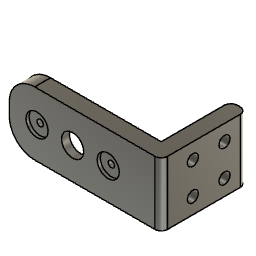
arm_1 v8 (Autodesk Fusion 360 design; units mm, degrees)
Autodesk Fusion 360 part; units mm, degrees
note: some values were not read from the file. Chosen so that the rebuilt part matches the saved one: which face or edge a step refers to.
sketch "스케치1" plane through (0, 0, 0) normal (0, 0, 1) x (1, 0, 0)
  line L0 (0, 0) -> (-45, 0)
  line L1 (-45, 0) -> (-45, 5)
  line L2 (-45, 5) -> (-5, 5)
  line L3 (0, 5) -> (0, 0)
  line L4 (0, 0) -> (-5, 0)
  line L5 (-5, 5) -> (-5, 30)
  line L6 (-5, 30) -> (0, 30)
  line L7 (0, 30) -> (0, 0)
  constraint horizontal L0
  constraint vertical L1
  constraint horizontal L2
  constraint vertical L3
  constraint coincident L0.start L3.end
  constraint horizontal L4
  constraint vertical L5
  constraint horizontal L6
  constraint vertical L7
extrude "돌출1" add sketch "스케치1" along normal blind 30
sketch "스케치2" plane through (0, 5, 0) normal (0, 1, 0) x (-1, 0, 0)
  circle A0 centre (25, 15) radius 7.5
  dimension "d3" = 15
  measures "d3" diameter of A0
extrude "돌출2" cut sketch "스케치2" against normal blind 2.5
sketch "스케치3" plane through (0, 5, 0) normal (0, 1, 0) x (-1, 0, 0)
  circle A0 centre (25, 15) radius 3.5
  dimension "d7" = 7
  measures "d7" diameter of A0
extrude "돌출3" cut sketch "스케치3" against normal blind 2.5 from surface at -2.5
sketch "스케치4" plane through (0, 5, 0) normal (0, 1, 0) x (-1, 0, 0)
sketch "스케치5" plane through (0, 0, 0) normal (0, -1, 0) x (1, 0, 0)
  circle A0 centre (-16.225, 15) radius 1
  dimension "d12" = 2
  measures "d12" diameter of A0
hole "구멍1" at (-16.225, 0, 15) direction (0, 1, 0) diameter 2 depth 7 tip angle 118
sketch "스케치6" plane through (0, 0, 0) normal (0, -1, 0) x (1, 0, 0)
hole "구멍2" at (-36.2538, 0, 15.3762) direction (0, 1, 0) diameter 2 depth 7 tip angle 118
delete_face "면 삭제1" 1 faces at (-16.1752, 1.6667, 14.0012)
sketch "스케치7" plane through (0, 0, 0) normal (0, -1, 0) x (1, 0, 0)
  circle A0 centre (-13.75, 15) radius 1
  dimension "d20" = 2
  measures "d20" diameter of A0
hole "구멍3" at (-13.75, 0, 15) direction (0, 1, 0) diameter 2 depth 7 tip angle 118
sketch "스케치8" plane through (0, 0, 0) normal (0, -1, 0) x (1, 0, 0)
delete_face "면 삭제2" 1 faces at (-35.9118, 1.6667, 16.3159)
delete_face "면 삭제3" 1 faces at (-13.7002, 1.6667, 14.0012)
sketch "스케치9" plane through (0, 0, 0) normal (0, -1, 0) x (1, 0, 0)
  circle A0 centre (-13.75, 15) radius 1
  dimension "d24" = 2
  measures "d24" diameter of A0
hole "구멍4" at (-13.75, 0, 15) direction (0, 1, 0) diameter 2 depth 7 tip angle 118
sketch "스케치10" plane through (0, 0, 0) normal (0, -1, 0) x (1, 0, 0)
  circle A0 centre (-36.25, 15) radius 1
  dimension "d28" = 2
  measures "d28" diameter of A0
hole "구멍5" at (-36.25, 0, 15) direction (0, 1, 0) diameter 2 depth 7 tip angle 118
sketch "스케치11" plane through (0, 0, 0) normal (0, -1, 0) x (1, 0, 0)
sketch "스케치12" plane through (0, 0, 0) normal (0, -1, 0) x (1, 0, 0)
sketch "스케치13" plane through (0, 0, 0) normal (0, -1, 0) x (1, 0, 0)
  circle A0 centre (-13.75, 15) radius 1
  circle A1 centre (-13.75, 15) radius 3.5
  dimension "d32" = 2
  dimension "d33" = 7
  constraint concentric A0 A1
  measures "d32" diameter of A0
  measures "d33" diameter of A1
extrude "돌출4" cut sketch "스케치13" against normal blind 1
sketch "스케치14" plane through (0, 0, 0) normal (0, -1, 0) x (1, 0, 0)
  circle A0 centre (-36.25, 15) radius 1
  circle A1 centre (-36.25, 15) radius 3.5
  dimension "d36" = 2
  dimension "d37" = 7
  constraint concentric A0 A1
  measures "d36" diameter of A0
  measures "d37" diameter of A1
extrude "돌출5" cut sketch "스케치14" against normal blind 1
sketch "스케치15" plane through (0, 0, 0) normal (1, 0, 0) x (0, 1, 0)
  circle A0 centre (20, 10) radius 1.75
  circle A1 centre (10, 10) radius 1.75
  circle A2 centre (20, 20) radius 1.75
  circle A3 centre (10, 20) radius 1.75
  dimension "d40" = 3.5
  dimension "d41" = 3.5
  dimension "d42" = 3.5
  dimension "d43" = 3.5
  measures "d40" diameter of A0
  measures "d41" diameter of A1
  measures "d42" diameter of A2
  measures "d43" diameter of A3
hole "구멍6" at (0, 20, 10) direction (-1, 0, 0) diameter 3.5 depth 7 tip angle 118
sketch "스케치16" plane through (0, 0, 0) normal (1, 0, 0) x (0, 1, 0)
  circle A0 centre (10, 10) radius 1.75
  dimension "d47" = 3.5
  measures "d47" diameter of A0
hole "구멍7" at (0, 10, 10) direction (-1, 0, 0) diameter 3.5 depth 7 tip angle 118
sketch "스케치17" plane through (0, 0, 0) normal (1, 0, 0) x (0, 1, 0)
  circle A0 centre (20, 20) radius 1.75
  dimension "d51" = 3.5
  measures "d51" diameter of A0
extrude "돌출6" cut sketch "스케치17" against normal blind 5
sketch "스케치18" plane through (0, 0, 0) normal (1, 0, 0) x (0, 1, 0)
  circle A0 centre (10, 20) radius 1.75
  dimension "d54" = 3.5
  measures "d54" diameter of A0
hole "구멍8" at (0, 10, 20) direction (-1, 0, 0) diameter 3.5 depth 7 tip angle 118
sketch "스케치19" plane through (0, 30, 0) normal (0, 1, 0) x (-1, 0, 0)
sketch "스케치20" plane through (0, 30, 0) normal (0, 1, 0) x (-1, 0, 0)
move_face "면 이동1" by (0, 0, 5) 1 faces at (-16.6667, 1.6667, 0)
move_face "면 이동2" by (0, 0, -5) 1 faces at (-16.6667, 1.6667, 30)
sketch "스케치24" plane through (0, 30, 0) normal (0, 1, 0) x (-1, 0, 0)
extrude "돌출7" cut 1 faces at (-3.3333, 30, 18.3333) along direction (0, -1, 0) blind 3
move_face "면 이동3" to x (1, 0, 0) y (0, 1, 0) z (0, 0, 1) at (-3, 0, 0) 3 faces at (-36.7283, 2.3333, 15.8782) (-33.5973, 1, 14.8012) (-32.7544, 0.6667, 14.8255)
move_face "면 이동4" to x (1, 0, 0) y (0, 1, 0) z (0, 0, 1) at (-3, 0, 0) 3 faces at (-28.4826, 0.8333, 14.6515) (-31.1257, 2.5, 14.4535) (-32.4907, 3.3333, 14.6262)
move_face "면 이동5" by (-3, 0, 0) 1 faces at (-45, 1.6667, 18.3333)
move_face "면 이동6" to x (1, 0, 0) y (0, 1, 0) z (0, 0, 1) at (-3, 0, 0) 3 faces at (-13.7002, 2.3333, 14.0012) (-11.0973, 1, 14.8012) (-10.2544, 0.6667, 14.8255)
fillet "모깎기6" radius 8 1 edges at (-48, 2.5, 25)
fillet "모깎기7" radius 8 1 edges at (-48, 2.5, 5)
fillet "모깎기8" radius 2 1 edges at (-5, 27, 15)
fillet "모깎기9" radius 2 1 edges at (0, 27, 15)
fillet "모깎기10" radius 2 1 edges at (0, 0, 15)
sketch "스케치25" plane through (0, 5, 0) normal (0, 1, 0) x (-1, 0, 0)
fillet "모깎기1" [suppressed]
fillet "모깎기2" [suppressed]
fillet "모깎기3" [suppressed]
fillet "모깎기4" [suppressed]
fillet "모깎기5" [suppressed]
sketch "스케치21" plane through (0, 5, 0) normal (0, 1, 0) x (-1, 0, 0)
  circle A0 centre (25, 15) radius 7.5
  circle A1 centre (25, 15) radius 3.5
  circle A2 centre (13.75, 15) radius 1
  circle A3 centre (36.25, 15) radius 1
  dimension "d68" = 15
  dimension "d69" = 7
  dimension "d70" = 2
  dimension "d71" = 2
  dimension "d72" = 11.25
  dimension "d73" = 11.25
  measures "d68" diameter of A0
  measures "d69" diameter of A1
  measures "d70" diameter of A2
  measures "d71" diameter of A3
  measures "d72" distance of A0.centre A3.centre
  measures "d73" distance of A0.centre A2.centre
sketch "스케치22" plane through (-45, 0, 0) normal (-1, 0, 0) x (0, -1, 0)
sketch "스케치23" plane through (0, 5, 0) normal (0, 1, 0) x (-1, 0, 0)
  circle A0 centre (36.25, 15) radius 1
  circle A1 centre (25, 15) radius 7.5
  circle A2 centre (25, 15) radius 3.5
  dimension "d74" = 2
  dimension "d75" = 15
  dimension "d76" = 7
  dimension "d77" = 11.25
  measures "d74" diameter of A0
  measures "d75" diameter of A1
  measures "d76" diameter of A2
  measures "d77" distance of A0.centre A1.centre
